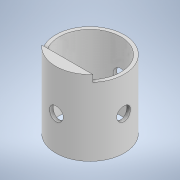
# Autodesk Inventor part: aiirframe
Saved by Autodesk Inventor 2022 (Build 260153000, 153)
## iProperties
Created: 2021-09-22
Part Number: aiirframe
Material: Generic
Document SubType Name: Modeling
Designer: WASHINGTON
Density: 1 g/cm^3
Appearance: Default
Author: WASHINGTON
Autodesk Inventor part; units mm, degrees
ref_plane "YZ Plane" through (0, 0, 0) normal (1, 0, 0) x (0, 1, 0)
ref_plane "XZ Plane" through (0, 0, 0) normal (0, 1, 0) x (-1, 0, 0)
ref_plane "XY Plane" through (0, 0, 0) normal (0, 0, 1) x (1, 0, 0)
sketch "Sketch1" plane through (0, 0, 0) normal (0, 1, 0) x (-1, 0, 0)
  circle A0 centre (0, 0) radius 22.5
  circle A1 centre (0, 0) radius 25
  dimension "d0" = 45
  dimension "d1" = 50
  constraints: 2 centre point, 2 coincident
  measures "d0" diameter of A0
  measures "d1" diameter of A1
extrude "Extrusion1" add sketch "Sketch1" along normal mid plane 50
sketch "Sketch2" plane through (0, 25, 0) normal (0, 1, 0) x (1, 0, 0)
  circle A0 centre (0, 0) radius 25 projected
  line L0 (-12.5, -21.6506) -> (12.5, -21.6506) construction
  line L1 (12.5, -21.6506) -> (12.5, -16.6506) construction
  line L2 (12.5, -16.6506) -> (-12.5, -16.6506)
  line L3 (-12.5, -16.6506) -> (-12.5, -21.6506) construction
  line L4 (12.5, -16.6506) -> (18.6482, -16.6506)
  line L5 (-12.5, -16.6506) -> (-18.6482, -16.6506)
  arc A1 (-18.6482, -16.6506) -> (18.6482, -16.6506) centre (0, 0) ccw
  dimension "d4" = 25
  dimension "d5" = 12.5
  dimension "d6" = 5
  dimension "d7" = 16.6506
  constraints: 12 end point, 5 point on circle, 2 horizontal, 2 parallel, 1 centre point, 1 coincident, 1 perpendicular, 1 point on line
  measures "d4" distance of L0.end L0.start
  measures "d5" horizontal distance of point (0, 0) L0.start
  measures "d6" distance of L2.end L0.start
  measures "d7" distance from line of A0.centre L4
extrude "Extrusion2" add sketch "Sketch2" along normal blind 5 contours L5 L2 L4 A0 picked at (-0.9999, -19.3735)
sketch "Sketch3" plane through (0, 0, 0) normal (0, 0, 1) x (1, 0, 0)
  circle A0 centre (0, 0) radius 5
  dimension "d10" = 10
  constraints: 1 centre point, 1 coincident
  measures "d10" diameter of A0
extrude "Extrusion3" cut sketch "Sketch3" along normal through all both and the other way through all
sketch "Sketch4" plane through (0, 0, 0) normal (1, 0, 0) x (0, 1, 0)
  circle A0 centre (0, 0) radius 5
  dimension "d13" = 10
  constraints: 1 centre point, 1 coincident
  measures "d13" diameter of A0
extrude "Extrusion4" cut sketch "Sketch4" along normal through all both and the other way through all
body "Solid1"
